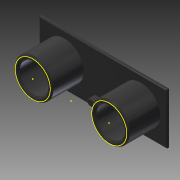
# Autodesk Inventor part: czujnik_ultra_dzwiek
Saved by Autodesk Inventor 2014 (Build 180170000, 170)
## iProperties
Created: 2013-10-18
Part Number: czujnik_ultra_dzwiek
Material: Kauczuk, silikon
Document SubType Name: Modeling
Designer: Wojciech
Density: 1.25 g/cm^3
Appearance: Kauczuk - czarny - wersja 1.1
Author: Wojciech
Autodesk Inventor part; units mm, degrees
ref_plane "YZ Plane" through (0, 0, 0) normal (1, 0, 0) x (0, 1, 0)
ref_plane "XZ Plane" through (0, 0, 0) normal (0, 1, 0) x (-1, 0, 0)
ref_plane "XY Plane" through (0, 0, 0) normal (0, 0, 1) x (1, 0, 0)
sketch "Szkic1" plane through (0, 0, 0) normal (0, 1, 0) x (-1, 0, 0)
  line L0 (-20, -8) -> (20, -8)
  line L1 (20, -8) -> (20, 8)
  line L2 (20, 8) -> (-20, 8)
  line L3 (-20, 8) -> (-20, -8)
  line L4 (-20, -8) -> (20, 8) construction
  line L5 (20, -8) -> (-20, 8) construction
  point P0 (0, 0)
  dimension "d0" = 40
  dimension "d1" = 16
  constraints: 12 end point, 2 midpoint, 2 parallel, 1 horizontal, 1 perpendicular
  measures "d0" distance of L2.end L1.end
  measures "d1" distance of L1.end L0.end
extrude "Wyciągnięcie proste1" add sketch "Szkic1" along normal blind 1
sketch "Szkic2" plane through (0, 0, 0) normal (0, -1, 0) x (1, 0, 0)
  circle A0 centre (-12, 0) radius 6
  circle A1 centre (12, 0) radius 6
  point P0 (0, 0)
  dimension "d4" = 12
  dimension "d5" = 12
  constraints: 2 centre point
  measures "d4" diameter of A0
  measures "d5" diameter of A1
extrude "Wyciągnięcie proste2" add sketch "Szkic2" along normal blind 10
sketch "Szkic3" plane through (0, 0, 0) normal (0, -1, 0) x (1, 0, 0)
  line L0 (20, -8) -> (-20, -8) projected
  line L1 (2, -5.5) -> (-2, -5.5) construction
  line L2 (2, -4.5) -> (-2, -4.5)
  line L3 (-2, -6.5) -> (2, -6.5)
  arc A0 (2, -6.5) -> (2, -4.5) centre (2, -5.5) ccw
  arc A1 (-2, -4.5) -> (-2, -6.5) centre (-2, -5.5) ccw
  point P0 (0, 0)
  point P1 (0, -5.5)
  dimension "d8" = 4
  dimension "d9" = 2
  constraints: 8 end point, 4 point on circle, 4 tangent, 2 centre point, 2 parallel, 1 midpoint
  measures "d8" distance of L1.start L1.end
  measures "d9" diameter of A1
extrude "Wyciągnięcie proste3" add sketch "Szkic3" along normal blind 2
chamfer "Faza1" distance 0.5 angle 45 1 edges at (-18, -10, 0)
chamfer "Faza2" distance 0.5 angle 45 1 edges at (6, -10, 0)
chamfer "Faza3" distance 0.2 angle 45 4 edges at (0, -2, -6.5) (3, -2, -5.5) (0, -2, -4.5) (-3, -2, -5.5)
chamfer "Faza4" distance 0.2 angle 45 1 edges at (0, 0, 8)
chamfer "Faza5" distance 0.2 angle 45 1 edges at (-20, 0, -0.1)
chamfer "Faza6" distance 0.2 angle 45 1 edges at (0.1, 0, -8)
chamfer "Faza7" distance 0.2 angle 45 1 edges at (20, 0, 0)
chamfer "Faza8" distance 0.2 angle 45 1 edges at (0, 1, 8)
chamfer "Faza9" distance 0.2 angle 45 1 edges at (20, 1, -0.1)
chamfer "Faza10" distance 0.2 angle 45 1 edges at (-0.1, 1, -8)
chamfer "Faza11" distance 0.2 angle 45 1 edges at (-20, 1, 0)
sketch "Szkic4" plane through (0, 1, 0) normal (0, 1, 0) x (1, 0, 0)
  line L0 (-17.7792, 4.1723) -> (-14.2918, 4.1723)
  line L1 (-14.2918, 4.1723) -> (-14.2918, -3.3005)
  line L2 (-14.2918, -3.3005) -> (-17.7792, -3.3005)
  line L3 (-17.7792, -3.3005) -> (-17.7792, 4.1723)
  line L4 (-17.7792, 4.1723) -> (-14.2918, -3.3005) construction
  line L5 (-14.2918, 4.1723) -> (-17.7792, -3.3005) construction
  line L6 (-9.9327, 3.7987) -> (-1.9616, 3.7987)
  line L7 (-1.9616, 3.7987) -> (-1.9616, -0.4359)
  line L8 (-1.9616, -0.4359) -> (-9.9327, -0.4359)
  line L9 (-9.9327, -0.4359) -> (-9.9327, 3.7987)
  line L10 (-9.9327, 3.7987) -> (-1.9616, -0.4359) construction
  line L11 (-1.9616, 3.7987) -> (-9.9327, -0.4359) construction
  line L12 (10.3063, -4.1101) -> (5.8226, -4.1101)
  line L13 (5.8226, -4.1101) -> (5.8226, 3.2382)
  line L14 (5.8226, 3.2382) -> (10.3063, 3.2382)
  line L15 (10.3063, 3.2382) -> (10.3063, -4.1101)
  line L16 (10.3063, -4.1101) -> (5.8226, 3.2382) construction
  line L17 (5.8226, -4.1101) -> (10.3063, 3.2382) construction
  point P0 (0, 0)
  point P1 (-16.0355, 0.4359)
  point P2 (-5.9471, 1.6814)
  point P3 (8.0645, -0.4359)
  constraints: 36 end point, 6 midpoint, 6 parallel, 3 horizontal, 3 perpendicular
extrude "Wyciągnięcie proste4" add sketch "Szkic4" along normal blind 1
chamfer "Faza12" distance 0.2 angle 45 13 edges at (-5.9471, 2, 0.4359) (-1.9616, 2, -1.6814) (-5.9471, 2, -3.7987) (-9.9327, 2, -1.6814) (-14.2918, 2, -0.4359) (-16.0355, 2, 3.3005) (-17.7792, 2, -0.4359) (-16.0355, 2, -4.1723) (8.0645, 2, 4.1101) (5.8226, 1, 0.4359) (10.3063, 2, 0.4359) (8.0645, 2, -3.2382) (5.8226, 2, 0.4359)
sketch "Szkic5" plane through (-12, -10, 0) normal (0, -1, 0) x (1, 0, 0)
  circle A0 centre (0, 0) radius 5.5 projected
  circle A1 centre (24, 0) radius 5.5 projected
  point P0 (12, 0)
sketch "Szkic6" plane through (-12, -10, 0) normal (0, -1, 0) x (1, 0, 0)
  circle A0 centre (0, 0) radius 5.5 projected
  circle A1 centre (0, 0) radius 4.5
  point P0 (12, 0)
  dimension "d50" = 9
  constraints: 1 centre point, 1 coincident
  measures "d50" diameter of A1
extrude "Wyciągnięcie proste5" cut sketch "Szkic6" against normal blind 7 contours A1
chamfer "Faza13" distance 0.5 angle 45 1 edges at (-16.5, -10, 0)
sketch "Szkic7" plane through (12, -10, 0) normal (0, -1, 0) x (1, 0, 0)
  circle A0 centre (0, 0) radius 5.5 projected
  circle A1 centre (0, 0) radius 4.5
  point P0 (-12, 0)
  dimension "d56" = 9
  constraints: 1 centre point, 1 coincident
  measures "d56" diameter of A1
extrude "Wyciągnięcie proste6" cut sketch "Szkic7" against normal blind 7 contours A1
chamfer "Faza14" distance 0.5 angle 45 1 edges at (7.5, -10, 0)
